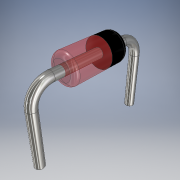
# Autodesk Inventor part: Diode
Saved by Autodesk Inventor 2018 (Build 220112000, 112)
## iProperties
Created: 2021-02-20
Part Number: Diode
Material: SAN plast
Document SubType Name: Modeling
Designer: Jozko Mrkvicka
Density: 1.068 g/cm^3
Appearance: Polykarbonát – čirý
Author: Jozko Mrkvicka
Autodesk Inventor part; units mm, degrees
sketch "Náčrt1" plane through (0, 0, 0) normal (0, 1, 0) x (-1, 0, 0)
  circle A0 centre (0, 0) radius 0.9525
  dimension "d0" = 1.905
  constraints: 1 centre point, 1 coincident
  measures "d0" diameter of A0
extrude "Vysunutí1" add sketch "Náčrt1" along normal blind 3.81
fillet "Zaoblení1" radius 0.3175 2 edges at (0.9525, 3.81, 0) (0.9525, 0, 0)
ref_plane "Pracovní rovina1" through (0, 1.27, 0) normal (0, -1, 0) x (1, 0, 0)
sketch "Náčrt2" plane through (0, 3.81, 0) normal (0, 1, 0) x (1, 0, 0)
  circle A0 centre (0, 0) radius 0.635 projected
  circle A1 centre (0, 0) radius 0.3175
  dimension "d5" = 0.635
  constraints: 1 centre point, 1 coincident
  measures "d5" diameter of A1
extrude "Vysunutí2" cut sketch "Náčrt2" against normal up to next contours A1
split body "Rozdělit1" result two bodies by plane through (0, 1.27, 0) normal (0, -1, 0) first body at (-0.4466, 0.9525, 0.0726)
sketch "Náčrt3" plane through (0, 3.81, 0) normal (0, 1, 0) x (1, 0, 0)
  circle A0 centre (0, 0) radius 0.3175 projected
extrude "Vysunutí3" add sketch "Náčrt3" along normal blind 5.08 bodies 3
ref_plane "Pracovní rovina2" through (0, 3.81, 0) normal (0, 1, 0) x (1, 0, 0)
split body "Rozdělit2" result two bodies by plane through (0, 3.81, 0) normal (0, 1, 0) bodies 3 first body at (-0.1819, 7.1967, -0.0147)
move or copy body "Posunout těleso1" bodies to move or copy 4 copy no translate (0, -4.445, 0)
ref_plane "Pracovní rovina3" through (0.3175, 4.445, 0) normal (0, 0, -1) x (-1, 0, 0)
sketch "Náčrt5" plane through (0.3175, 4.445, 0) normal (0, 0, -1) x (-1, 0, 0)
  line L0 (0.635, 0) -> (0, 0) projected
  line L1 (1.5875, 1.27) -> (5.3975, 1.27)
  line L2 (0, -5.08) -> (0.635, -5.08) projected
  line L3 (1.5875, -6.35) -> (5.3975, -6.35)
  arc A0 (1.5875, 1.27) -> (0.3175, 0) centre (1.5875, 0) ccw
  line L4 (0.3175, 0) -> (1.5875, 1.27) construction
  line L5 (0.3175, 0) -> (2.1136, 0) construction
  arc A1 (0.3175, -5.08) -> (1.5875, -6.35) centre (1.5875, -5.08) ccw
  point P0 (0.3175, -4.445)
  dimension "d18" = 45
  dimension "d19" = 1.27
  dimension "d20" = 1.27
  constraints: 8 end point, 4 point on circle, 2 centre point, 2 midpoint, 1 equal length, 1 horizontal
  measures "d18" angle of L5 L4
  measures "d19" radius of A0
  measures "d20" radius of A1
sketch "Náčrt6" plane through (0, -0.635, 0) normal (0, -1, 0) x (1, 0, 0)
  circle A0 centre (0, 0) radius 0.3175 projected
sketch "Náčrt7" plane through (0, 4.445, 0) normal (0, 1, 0) x (1, 0, 0)
  circle A0 centre (0, 0) radius 0.3175 projected
sweep "Tažení1" add profiles "Náčrt7" path "Náčrt5" bodies 4 path curves A0 L1
sweep "Tažení2" add profiles "Náčrt6" path "Náčrt5" bodies 4 path curves A1 L3
